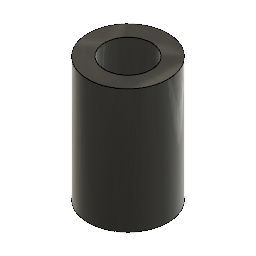
Pneumatics Module 2 (Autodesk Fusion 360 archive; units mm, degrees)
design "CIS-PM-005 0.367 in Angle Spacer v2"
Autodesk Fusion 360 part; units mm, degrees
sketch "Sketch1" plane through (0, 0, 0) normal (0, 1, 0) x (1, 0, 0)
  circle A0 centre (0, 0) radius 1.75
  circle A1 centre (0, 0) radius 3
  dimension "d1" = 3.5
  dimension "d2" = 6
  measures "d1" diameter of A0
  measures "d2" diameter of A1
extrude "Extrude1" add sketch "Sketch1" along normal blind 5.08
extrude "Extrude2" add 1 faces at (2.5656, 5.08, 0.236) along direction (0, 1, 0) blind 9.3218
extrude "Extrude3" cut 1 faces at (2.5656, 14.4018, 0.236) along direction (0, -1, 0) blind 5.08

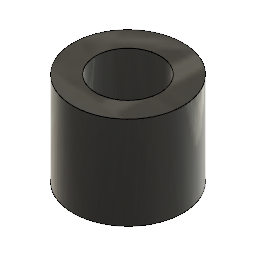
design "CIS-PM-002 .2in Spacer"
Autodesk Fusion 360 part; units mm, degrees
sketch "Sketch1" plane through (0, 0, 0) normal (0, 1, 0) x (1, 0, 0)
  circle A0 centre (0, 0) radius 1.75
  circle A1 centre (0, 0) radius 3
  dimension "d1" = 3.5
  dimension "d2" = 6
  measures "d1" diameter of A0
  measures "d2" diameter of A1
extrude "Extrude1" add sketch "Sketch1" along normal blind 5.08

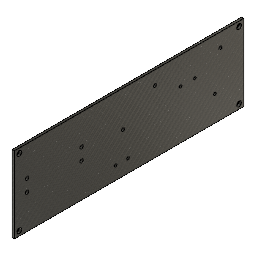
design "Pneumatics Module Plate 2"
Autodesk Fusion 360 part; units mm, degrees
sketch "Sketch1" plane through (0, 0, 0) normal (1, 0, 0) x (0, 1, 0)
  line L0 (152.4, -50.8) -> (-152.4, -50.8)
  line L1 (-152.4, -50.8) -> (-152.4, 50.8)
  line L2 (-152.4, 50.8) -> (152.4, 50.8)
  line L3 (152.4, 50.8) -> (152.4, -50.8)
  line L4 (152.4, -50.8) -> (-152.4, 50.8) construction
  line L5 (-152.4, -50.8) -> (152.4, 50.8) construction
  dimension "d46" = 101.6
  dimension "d47" = 304.8
extrude "Extrude1" add sketch "Sketch1" along normal mid plane 3.175
sketch "Sketch2" plane through (1.5875, 0, 0) normal (1, 0, 0) x (0, 1, 0)
  line L0 (152.4, 50.8) -> (-152.4, 50.8)
  line L1 (-152.4, 50.8) -> (-152.4, -50.8)
  line L2 (-152.4, -50.8) -> (152.4, -50.8)
  line L3 (152.4, -50.8) -> (152.4, 50.8)
  circle A0 centre (-146.05, 44.45) radius 3.175
  circle A1 centre (-146.05, -44.45) radius 3.175
  circle A2 centre (146.05, -44.45) radius 3.175
  circle A3 centre (146.05, 44.45) radius 3.175
  dimension "d7" = 6.35
  dimension "d8" = 6.35
  dimension "d9" = 6.35
  dimension "d10" = 6.35
  dimension "d38" = 6.35
  dimension "d39" = 6.35
  dimension "d40" = 6.35
  dimension "d41" = 6.35
  dimension "d42" = 6.35
  dimension "d43" = 6.35
  dimension "d44" = 6.35
  dimension "d45" = 6.35
  measures "d7" diameter of A0
  measures "d8" diameter of A1
  measures "d9" diameter of A2
  measures "d10" diameter of A3
extrude "Extrude2" cut sketch "Sketch2" against normal blind 38.1 contours A0 | A1 | A2 | A3
sketch "Sketch3" plane through (1.5875, 0, 0) normal (1, 0, 0) x (0, 1, 0)
  circle A0 centre (146.05, 44.45) radius 3.175
  circle A1 centre (-146.05, -44.45) radius 3.175
  circle A2 centre (-146.05, 44.45) radius 3.175
  circle A3 centre (146.05, -44.45) radius 3.175
  line L0 (152.4, 50.8) -> (-152.4, 50.8)
  line L1 (-152.4, 50.8) -> (-152.4, -50.8)
  line L2 (-152.4, -50.8) -> (152.4, -50.8)
  line L3 (152.4, -50.8) -> (152.4, 50.8)
  line L4 (-135.7, 10.65) -> (-63.2, 10.65) construction
  line L5 (-63.2, 10.65) -> (-63.2, -5.35) construction
  line L6 (-63.2, -5.35) -> (-135.7, -5.35) construction
  line L7 (-135.7, -5.35) -> (-135.7, 10.65) construction
  line L8 (-139.7, 15.85) -> (-59.2, 15.85) construction
  line L9 (-59.2, 15.85) -> (-59.2, -15.85) construction
  line L10 (-59.2, -15.85) -> (-139.7, -15.85) construction
  line L11 (-139.7, -15.85) -> (-139.7, 15.85) construction
  line L12 (-139.7, 0) -> (-59.2, 0) construction
  circle A4 centre (-135.7, -5.35) radius 2.25
  circle A5 centre (-63.2, -5.35) radius 2.25
  circle A6 centre (-63.2, 10.65) radius 2.25
  circle A7 centre (-135.7, 10.65) radius 2.25
  dimension "d13" = 72.5
  dimension "d14" = 16
  dimension "d15" = 80.5
  dimension "d16" = 31.7
  dimension "d18" = 4
  dimension "d19" = 12.7
  dimension "d21" = 4.5
  dimension "d22" = 4.5
  dimension "d23" = 4.5
  dimension "d24" = 4.5
  dimension "d25" = 10.5
  dimension "d49" = 50.8
  measures "d18" distance of L7 L11
  measures "d19" distance of L1 L11
  measures "d21" diameter of A4
  measures "d22" diameter of A5
  measures "d23" diameter of A6
  measures "d24" diameter of A7
  measures "d25" distance of L6 L10
  measures "d49" distance of L2 L12
extrude "Extrude3" cut sketch "Sketch3" against normal blind 7.62 contours A4 | A5 | A6 | A7
sketch "Sketch4" plane through (1.5875, 0, 0) normal (1, 0, 0) x (0, 1, 0)
  circle A0 centre (-135.7, -5.35) radius 2.25
  circle A1 centre (-63.2, -5.35) radius 2.25
  circle A2 centre (-135.7, 10.65) radius 2.25
  circle A3 centre (-63.2, 10.65) radius 2.25
  circle A4 centre (146.05, 44.45) radius 3.175
  circle A5 centre (-146.05, -44.45) radius 3.175
  circle A6 centre (-146.05, 44.45) radius 3.175
  circle A7 centre (146.05, -44.45) radius 3.175
  line L0 (152.4, 50.8) -> (-152.4, 50.8)
  line L1 (-152.4, 50.8) -> (-152.4, -50.8)
  line L2 (-152.4, -50.8) -> (152.4, -50.8)
  line L3 (152.4, -50.8) -> (152.4, 50.8)
  line L4 (-18.0594, -33.2994) -> (-1.5594, -33.2994)
  circle A8 centre (-18.0594, -33.2994) radius 1.75
  circle A9 centre (-1.5594, -33.2994) radius 1.75
  dimension "d28" = 16.5
  dimension "d29" = 3.5
  dimension "d30" = 3.5
  dimension "d33" = 134.3406
  dimension "d50" = 17.5006
  measures "d29" diameter of A8
  measures "d30" diameter of A9
extrude "Extrude4" cut sketch "Sketch4" against normal blind 7.62 contours A8 | A9
sketch "Sketch5" plane through (1.5875, 0, 0) normal (1, 0, 0) x (0, 1, 0)
  circle A0 centre (-1.5594, -33.2994) radius 1.75
  circle A1 centre (-18.0594, -33.2994) radius 1.75
  circle A2 centre (-135.7, -5.35) radius 2.25
  circle A3 centre (-63.2, -5.35) radius 2.25
  circle A4 centre (-135.7, 10.65) radius 2.25
  circle A5 centre (-63.2, 10.65) radius 2.25
  circle A6 centre (146.05, 44.45) radius 3.175
  circle A7 centre (-146.05, -44.45) radius 3.175
  circle A8 centre (-146.05, 44.45) radius 3.175
  circle A9 centre (146.05, -44.45) radius 3.175
  line L0 (152.4, 50.8) -> (-152.4, 50.8)
  line L1 (-152.4, 50.8) -> (-152.4, -50.8)
  line L2 (-152.4, -50.8) -> (152.4, -50.8)
  line L3 (152.4, -50.8) -> (152.4, 50.8)
  circle A10 centre (68.3006, 14.478) radius 1.7526
  circle A11 centre (87.2998, 14.478) radius 1.7526
  line L4 (68.3006, 14.478) -> (87.2998, 14.478)
  dimension "d51" = 3.5052
  dimension "d52" = 3.5052
  dimension "d53" = 18.9992
  dimension "d54" = 65.1002
  dimension "d55" = 65.278
  measures "d51" diameter of A10
  measures "d52" diameter of A11
extrude "Extrude5" cut sketch "Sketch5" against normal blind 15.24 contours A10 | A11
sketch "Sketch6" plane through (1.5875, 0, 0) normal (1, 0, 0) x (0, 1, 0)
  circle A0 centre (87.2998, 14.478) radius 1.7526
  circle A1 centre (68.3006, 14.478) radius 1.7526
  circle A2 centre (-1.5594, -33.2994) radius 1.75
  circle A3 centre (-18.0594, -33.2994) radius 1.75
  circle A4 centre (-135.7, -5.35) radius 2.25
  circle A5 centre (-63.2, -5.35) radius 2.25
  circle A6 centre (-135.7, 10.65) radius 2.25
  circle A7 centre (-63.2, 10.65) radius 2.25
  circle A8 centre (146.05, 44.45) radius 3.175
  circle A9 centre (-146.05, -44.45) radius 3.175
  circle A10 centre (-146.05, 44.45) radius 3.175
  circle A11 centre (146.05, -44.45) radius 3.175
  line L0 (152.4, 50.8) -> (-152.4, 50.8)
  line L1 (-152.4, 50.8) -> (-152.4, -50.8)
  line L2 (-152.4, -50.8) -> (152.4, -50.8)
  line L3 (152.4, -50.8) -> (152.4, 50.8)
  circle A12 centre (113.8936, -16.7894) radius 1.7526
  dimension "d58" = 3.5052
  dimension "d59" = 34.0106
  dimension "d60" = 38.5064
  measures "d58" diameter of A12
extrude "Extrude6" cut sketch "Sketch6" against normal blind 15.24 contours A12
sketch "Sketch7" plane through (1.5875, 0, 0) normal (1, 0, 0) x (0, 1, 0)
  circle A0 centre (113.8936, -16.7894) radius 1.7526
  circle A1 centre (87.2998, 14.478) radius 1.7526
  circle A2 centre (68.3006, 14.478) radius 1.7526
  circle A3 centre (-1.5594, -33.2994) radius 1.75
  circle A4 centre (-18.0594, -33.2994) radius 1.75
  circle A5 centre (-135.7, -5.35) radius 2.25
  circle A6 centre (-63.2, -5.35) radius 2.25
  circle A7 centre (-135.7, 10.65) radius 2.25
  circle A8 centre (-63.2, 10.65) radius 2.25
  circle A9 centre (146.05, 44.45) radius 3.175
  circle A10 centre (-146.05, -44.45) radius 3.175
  circle A11 centre (-146.05, 44.45) radius 3.175
  circle A12 centre (146.05, -44.45) radius 3.175
  line L0 (152.4, 50.8) -> (-152.4, 50.8)
  line L1 (-152.4, 50.8) -> (-152.4, -50.8)
  line L2 (-152.4, -50.8) -> (152.4, -50.8)
  line L3 (152.4, -50.8) -> (152.4, 50.8)
  circle A13 centre (121.285, 32.4866) radius 2.0447
  circle A14 centre (-8.1534, 2.9972) radius 2.0447
  dimension "d63" = 4.0894
  dimension "d64" = 4.0894
  dimension "d65" = 18.3134
  dimension "d66" = 31.115
  dimension "d67" = 160.5534
  dimension "d68" = 53.7972
  measures "d63" diameter of A13
  measures "d64" diameter of A14
extrude "Extrude7" cut sketch "Sketch7" against normal blind 15.24 contours A13 | A14
sketch "Sketch8" plane through (-1.5875, 0, 0) normal (-1, 0, 0) x (0, -1, 0)
  circle A0 centre (8.1534, 2.9972) radius 2.0447
  circle A1 centre (-121.285, 32.4866) radius 2.0447
  circle A2 centre (-113.8936, -16.7894) radius 1.7526
  circle A3 centre (-87.2998, 14.478) radius 1.7526
  circle A4 centre (-68.3006, 14.478) radius 1.7526
  circle A5 centre (1.5594, -33.2994) radius 1.75
  circle A6 centre (18.0594, -33.2994) radius 1.75
  circle A7 centre (135.7, -5.35) radius 2.25
  circle A8 centre (63.2, -5.35) radius 2.25
  circle A9 centre (135.7, 10.65) radius 2.25
  circle A10 centre (63.2, 10.65) radius 2.25
  circle A11 centre (-146.05, 44.45) radius 3.175
  circle A12 centre (146.05, -44.45) radius 3.175
  circle A13 centre (146.05, 44.45) radius 3.175
  circle A14 centre (-146.05, -44.45) radius 3.175
  line L0 (152.4, 50.8) -> (-152.4, 50.8)
  line L1 (-152.4, 50.8) -> (-152.4, -50.8)
  line L2 (-152.4, -50.8) -> (152.4, -50.8)
  line L3 (152.4, -50.8) -> (152.4, 50.8)
  circle A15 centre (-34.2646, 32.4866) radius 2.0447
  line L4 (-121.285, 32.4866) -> (21.9558, 32.4866)
  dimension "d71" = 4.0894
  dimension "d72" = 118.1354
  measures "d71" diameter of A15
extrude "Extrude8" cut sketch "Sketch8" against normal blind 5.08 contours A15 L4 | A15 L4
